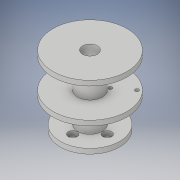
# Autodesk Inventor part: SpoolMk2
Saved by Autodesk Inventor 2019 (Build 230136000, 136)
## iProperties
Created: 2019-02-23
Part Number: SpoolMk2
Material: Generic
Document SubType Name: Modeling
Designer: Kepler
Density: 1 g/cm^3
Appearance: Default
Author: Kepler
Autodesk Inventor part; units mm, degrees
ref_plane "YZ Plane" through (0, 0, 0) normal (1, 0, 0) x (0, 1, 0)
ref_plane "XZ Plane" through (0, 0, 0) normal (0, 1, 0) x (-1, 0, 0)
ref_plane "XY Plane" through (0, 0, 0) normal (0, 0, 1) x (1, 0, 0)
sketch "Sketch1" plane through (0, 0, 0) normal (0, 0, 1) x (1, 0, 0)
  line L0 (0, 24) -> (0, 0)
  line L1 (3, 0) -> (3, 28)
  line L2 (3, 0) -> (12, 0)
  line L3 (12, 0) -> (12, 2)
  line L4 (12, 2) -> (5, 2)
  line L5 (5, 2) -> (5, 12)
  line L6 (5, 12) -> (15, 12)
  line L7 (15, 12) -> (15, 14)
  line L8 (15, 14) -> (5, 14)
  line L9 (5, 14) -> (5, 26)
  line L10 (5, 26) -> (15, 26)
  line L11 (15, 26) -> (15, 28)
  line L12 (15, 28) -> (3, 28)
  dimension "d1" = 6
  dimension "d2" = 9
  dimension "d3" = 2
  dimension "d4" = 7
  dimension "d5" = 2
  dimension "d6" = 10
  dimension "d7" = 2
  dimension "d8" = 2
  dimension "d9" = 28
  dimension "d10" = 12
  dimension "d11" = 10
  dimension "d17" = 26
  dimension "d18" = 2
  constraints: 26 end point, 8 perpendicular, 2 horizontal, 2 point on line, 1 collinear
  measures "d1" diameter of L1 L0
  measures "d2" distance of L1.start L2.end
  measures "d3" distance of L2.end L3.end
  measures "d4" distance of L3.end L4.end
  measures "d5" distance between parallel lines of L5 L1
  measures "d6" distance of L5.end L6.end
  measures "d7" distance of L6.end L7.end
  measures "d8" distance of L10.end L11.end
  measures "d9" distance between parallel lines of L2 L12
  measures "d10" distance between parallel lines of L8 L10
  measures "d11" distance between parallel lines of L4 L6
  measures "d17" distance from line of L0.end L10
  measures "d18" distance from line of L0.start L10
revolve "Revolution1" add sketch "Sketch1" angle 360 about axis through (0, 24, 0) along (0, -1, 0)
sketch "Sketch2" plane through (0, 0, 0) normal (0, -1, 0) x (1, 0, 0)
  circle A0 centre (0, -7) radius 1.8
  circle A1 centre (7, 0) radius 1.8
  circle A2 centre (0, 7) radius 1.8
  circle A3 centre (-7, 0) radius 1.8
  point P0 (0, 0)
  dimension "d20" = 3.6
  dimension "d21" = 7
  dimension "d24" = 360
  constraints: 4 centre point, 9 other
  measures "d20" diameter of A0
  measures "d21" distance of point (0, 0) A0.centre
extrude "Extrusion1" cut sketch "Sketch2" against normal blind 2
sketch "Sketch3" plane through (0, 12, 0) normal (0, -1, 0) x (1, 0, 0)
  point P0 (0, 0)
  point P1 (3.3947, -4.7826)
hole "Hole1" at (3.3947, 12, -4.7826) direction (0, 1, 0) diameter 1.5 depth 2
sketch "Sketch4" plane through (0, 12, 0) normal (0, -1, 0) x (1, 0, 0)
  point P0 (0, 0)
  point P1 (9.5617, -9.4421)
hole "Hole2" at (9.5617, 12, -9.4421) direction (0, 1, 0) diameter 1.5 depth 2
body "Solid1"
